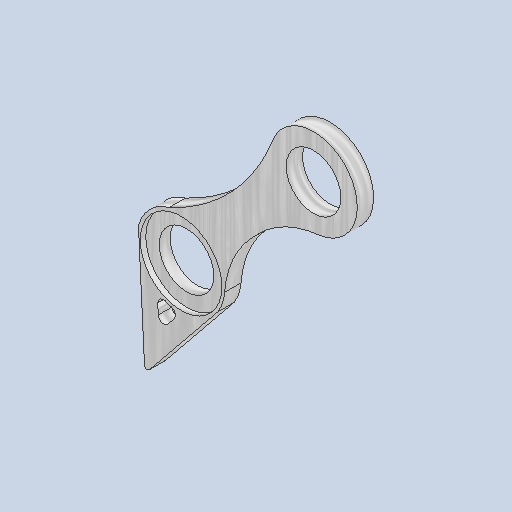
# Autodesk Inventor part: アーム 揺動節
Saved by Autodesk Inventor 2023 (Build 270158030, 158C)
## iProperties
Created: 2019-09-05
Part Number: アーム 揺動節
Material: アルミニウム 7075
Document SubType Name: Modeling
Designer: 雪村
Density: 2.81 g/cm^3
Appearance: サテン - ブラシ仕上げ 重厚
Mass: 3.77729 g
Surface Area: 16.4358 cm^2
Volume: 1.34423 cm^3
Description: アルミ2000 3t
Author: 雪村
Autodesk Inventor part; units mm, degrees
ref_plane "YZ Plane" through (0, 0, 0) normal (1, 0, 0) x (0, 1, 0)
ref_plane "XZ Plane" through (0, 0, 0) normal (0, 1, 0) x (-1, 0, 0)
ref_plane "XY Plane" through (0, 0, 0) normal (0, 0, 1) x (1, 0, 0)
sketch "スケッチ2" plane through (0, 0, 0) normal (0, 0, 1) x (1, 0, 0)
  circle A0 centre (-56.644, 91.4364) radius 8.025
  circle A1 centre (-56.644, 91.4364) radius 5.025
  arc A2 (-29.1424, 109.2011) -> (-49.1672, 88.5212) centre (-14.5297, 75.0161) ccw
  arc A3 (-59.7983, 98.8155) -> (-39.7735, 119.4954) centre (-74.411, 133.0005) ccw
  circle A4 centre (-32.2967, 116.5802) radius 8.025
  circle A5 centre (-32.2967, 116.5802) radius 5.025
  line L0 (-50.8789, 85.8539) -> (-64.3562, 71.9357)
  line L1 (-64.3562, 71.9357) -> (-64.668, 91.3073)
  line L2 (-56.644, 91.4364) -> (-32.2967, 116.5802) construction
  point P0 (0, 0)
  point P1 (0, 0)
  dimension "d5" = 45
  constraints: 6 centre point, 6 end point, 6 point on circle, 2 tangent, 1 parallel, 7 other
  measures "d5" angle of L0 L1
extrude "押し出し2" add sketch "スケッチ2" along normal blind 3
fillet "フィレット2" radius 0.5 1 edges at (-64.3562, 71.9357, 1.5)
sketch "スケッチ3" plane through (0, 0, 3) normal (0, 0, 1) x (1, 0, 0)
  line L0 (-63.5165, 72.8029) -> (-50.8789, 85.8539) projected
  arc A0 (-64.3756, 73.1427) -> (-63.5165, 72.8029) centre (-63.8757, 73.1507) ccw projected
  line L1 (-64.668, 91.3073) -> (-64.3756, 73.1427) projected
  arc A1 (-59.7983, 98.8155) -> (-64.668, 91.3073) centre (-56.644, 91.4364) ccw projected
  circle A2 centre (-56.644, 91.4364) radius 5.025 projected
  arc A3 (-50.8789, 85.8539) -> (-49.1672, 88.5212) centre (-56.644, 91.4364) ccw projected
  line L2 (-64.2129, 94.1033) -> (-63.8416, 71.0319)
  point P0 (0, 0)
  point P1 (-63.8676, 72.6508)
  dimension "d9" = 0.5
  constraints: 2 end point, 1 parallel, 1 point on circle
  measures "d9" distance between parallel lines of L1 L2
extrude "押し出し3" cut sketch "スケッチ3" against normal through all
fillet "フィレット3" radius 1 1 edges at (-63.8676, 72.6508, 1.5)
sketch "スケッチ4" plane through (0, 0, 3) normal (0, 0, 1) x (1, 0, 0)
  circle A0 centre (-56.644, 91.4364) radius 5.025 projected
  circle A1 centre (-32.2967, 116.5802) radius 5.025 projected
  arc A2 (-50.8789, 85.8539) -> (-49.1672, 88.5212) centre (-56.644, 91.4364) ccw projected
  line L0 (-50.8789, 85.8539) -> (-62.1849, 74.178) projected
  arc A3 (-63.9031, 74.8576) -> (-62.1849, 74.178) centre (-62.9033, 74.8737) ccw projected
  line L1 (-63.9031, 74.8576) -> (-64.2129, 94.1033) projected
  arc A4 (-59.7983, 98.8155) -> (-64.2129, 94.1033) centre (-56.644, 91.4364) ccw projected
  arc A5 (-59.7983, 98.8155) -> (-39.7735, 119.4954) centre (-74.411, 133.0005) ccw projected
  arc A6 (-29.1424, 109.2011) -> (-39.7735, 119.4954) centre (-32.2967, 116.5802) ccw projected
  arc A7 (-29.1424, 109.2011) -> (-49.1672, 88.5212) centre (-14.5297, 75.0161) ccw projected
  point P0 (0, 0)
sketch "スケッチ5" plane through (0, 0, 3) normal (0, 0, 1) x (1, 0, 0)
  circle A0 centre (-56.6451, 91.4352) radius 5.025
  circle A1 centre (-32.2979, 116.579) radius 5.025
  arc A2 (-50.2754, 86.5539) -> (-49.1683, 88.52) centre (-56.6451, 91.4352) ccw
  line L0 (-53.8399, 82.796) -> (-62.186, 74.1768)
  arc A3 (-63.9043, 74.8564) -> (-63.4923, 74.0635) centre (-62.9044, 74.8725) ccw
  line L1 (-63.9043, 74.8564) -> (-64.1215, 88.3503)
  arc A4 (-59.7994, 98.8143) -> (-64.4699, 93.2166) centre (-56.6451, 91.4352) ccw
  arc A5 (-59.7994, 98.8143) -> (-39.7746, 119.4942) centre (-74.4122, 132.9993) ccw
  arc A6 (-29.1436, 109.1999) -> (-39.7746, 119.4942) centre (-32.2979, 116.579) ccw
  arc A7 (-29.1436, 109.1999) -> (-49.1683, 88.52) centre (-14.5308, 75.0149) ccw
  line L2 (-83.3619, 46.2586) -> (-83.0117, 46.8656)
  arc A8 (-83.0117, 46.8656) -> (-84.2091, 48.3089) centre (-83.8778, 47.3654) ccw
  arc A9 (-84.8038, 48.1181) -> (-84.2091, 48.3089) centre (-88.0269, 59.1832) ccw
  arc A10 (-84.8038, 48.1181) -> (-85.306, 46.5345) centre (-84.5242, 47.158) ccw
  arc A11 (-85.0521, 46.1918) -> (-85.306, 46.5345) centre (-90.0169, 42.7785) ccw
  arc A12 (-85.0521, 46.1918) -> (-83.3619, 46.2586) centre (-84.2281, 46.7584) ccw
  arc A13 (-83.3002, 71.3425) -> (-83.1434, 69.6224) centre (-82.7197, 70.5282) ccw
  arc A14 (-76.5108, 59.6362) -> (-83.1434, 69.6224) centre (-88.0269, 59.1832) ccw
  arc A15 (-76.5108, 59.6362) -> (-74.7281, 59.0541) centre (-75.5116, 59.6755) ccw
  line L3 (-74.7281, 59.0541) -> (-66.7908, 69.0625)
  arc A16 (-66.7908, 69.0625) -> (-66.5756, 69.7348) centre (-67.5743, 69.6838) ccw
  line L4 (-66.5756, 69.7348) -> (-66.7153, 72.4721)
  arc A17 (-66.7153, 72.4721) -> (-67.8599, 73.4104) centre (-67.714, 72.4211) ccw
  arc A18 (-72.6132, 76.6262) -> (-67.8599, 73.4104) centre (-68.4798, 77.615) ccw
  arc A19 (-72.6132, 76.6262) -> (-73.9849, 77.3105) centre (-73.5858, 76.3936) ccw
  arc A20 (-73.9849, 77.3105) -> (-82.4826, 71.9828) centre (-60.5442, 46.4316) ccw
  arc A21 (-83.3002, 71.3425) -> (-82.4826, 71.9828) centre (-89.9903, 80.7269) ccw
  arc A22 (-110.8315, 31.539) -> (-109.4939, 30.5036) centre (-109.8361, 31.4432) ccw
  arc A23 (-101.7829, 26.9363) -> (-109.4939, 30.5036) centre (-107.4323, 24.8423) ccw
  arc A24 (-101.7829, 26.9363) -> (-100.1278, 26.5873) centre (-100.8452, 27.2839) ccw
  line L5 (-100.1278, 26.5873) -> (-91.546, 35.4257)
  arc A25 (-91.546, 35.4257) -> (-91.9436, 37.0698) centre (-92.2634, 36.1224) ccw
  arc A26 (-93.6931, 47.552) -> (-91.9436, 37.0698) centre (-90.0169, 42.7785) ccw
  arc A27 (-93.6931, 47.552) -> (-93.8022, 49.2096) centre (-94.3033, 48.3443) ccw
  arc A28 (-99.3351, 56.9581) -> (-93.8022, 49.2096) centre (-88.0269, 59.1832) ccw
  arc A29 (-99.3351, 56.9581) -> (-101.1863, 57.258) centre (-100.3162, 56.765) ccw
  line L6 (-101.1863, 57.258) -> (-106.2752, 48.2771)
  arc A30 (-106.2752, 48.2771) -> (-105.4755, 46.7866) centre (-105.4052, 47.7841) ccw
  arc A31 (-109.0024, 35.6122) -> (-105.4755, 46.7866) centre (-105.8991, 40.7765) ccw
  arc A32 (-109.0024, 35.6122) -> (-110.5128, 34.8508) centre (-109.5174, 34.755) ccw
  line L7 (-110.5128, 34.8508) -> (-110.8315, 31.539)
  circle A33 centre (-68.4798, 77.615) radius 1.25
  arc A34 (-64.1344, 80.7577) -> (-66.454, 82.6296) centre (-66.1318, 80.6557) ccw
  line L8 (-64.1344, 80.7577) -> (-63.5026, 68.3807)
  line L9 (-63.5026, 68.3807) -> (-76.8311, 51.5743)
  line L10 (-76.8311, 51.5743) -> (-83.9322, 39.2676)
  arc A35 (-84.9769, 37.8848) -> (-83.9322, 39.2676) centre (-90.0169, 42.7785) ccw
  line L11 (-84.9769, 37.8848) -> (-102.3922, 19.9486)
  arc A36 (-114.425, 25.5151) -> (-102.3922, 19.9486) centre (-107.4323, 24.8423) ccw
  line L12 (-114.425, 25.5151) -> (-112.8918, 41.4493)
  arc A37 (-112.0111, 44.2398) -> (-112.8918, 41.4493) centre (-105.8991, 40.7765) ccw
  line L13 (-112.0111, 44.2398) -> (-99.7723, 65.8386)
  arc A38 (-91.2432, 72.2945) -> (-99.7723, 65.8386) centre (-88.0269, 59.1832) ccw
  arc A39 (-91.2432, 72.2945) -> (-84.4369, 74.2589) centre (-89.9903, 80.7269) ccw
  arc A40 (-66.454, 82.6296) -> (-84.4369, 74.2589) centre (-60.5442, 46.4316) ccw
  circle A41 centre (-56.6793, 91.4683) radius 4
  circle A42 centre (-56.6793, 91.4683) radius 1.25
  circle A43 centre (-90.0169, 42.7785) radius 3.025
  circle A44 centre (-105.8991, 40.7765) radius 3.025
  circle A45 centre (-107.4323, 24.8423) radius 3.025
  circle A46 centre (-88.0269, 59.1832) radius 8.525
  circle A47 centre (-56.6793, 91.4683) radius 1.25
  line L14 (-32.2979, 116.579) -> (-56.6793, 91.4683)
  line L15 (-56.6793, 91.4683) -> (-88.0269, 59.1832)
  line L16 (-63.1972, 68.283) -> (-63.8347, 80.773)
  arc A48 (-63.8347, 80.773) -> (-66.5024, 82.9257) centre (-66.1318, 80.6557) ccw
  arc A49 (-66.5024, 82.9257) -> (-84.6323, 74.4865) centre (-60.5442, 46.4316) ccw
  arc A50 (-91.2565, 72.6) -> (-84.6323, 74.4865) centre (-89.9903, 80.7269) ccw
  arc A51 (-91.2565, 72.6) -> (-100.0334, 65.9865) centre (-88.0269, 59.1832) ccw
  line L17 (-100.0334, 65.9865) -> (-112.2721, 44.3877)
  arc A52 (-112.2721, 44.3877) -> (-113.1904, 41.4781) centre (-105.8991, 40.7765) ccw
  line L18 (-113.1904, 41.4781) -> (-114.7236, 25.5439)
  arc A53 (-114.7236, 25.5439) -> (-102.177, 19.7396) centre (-107.4323, 24.8423) ccw
  line L19 (-102.177, 19.7396) -> (-84.7616, 37.6758)
  arc A54 (-84.7616, 37.6758) -> (-83.6724, 39.1176) centre (-90.0169, 42.7785) ccw
  line L20 (-83.6724, 39.1176) -> (-76.5823, 51.4052)
  line L21 (-76.5823, 51.4052) -> (-63.1972, 68.283)
  arc A55 (-50.1385, 86.7434) -> (-64.1215, 88.3503) centre (-56.6793, 91.4683) ccw
  line L22 (-63.8347, 80.773) -> (-64.5039, 93.8831)
  line L23 (-76.8311, 51.5743) -> (-63.2204, 68.7366)
  circle A56 centre (-62.7886, 70.0857) radius 0.5
  line L24 (-62.3833, 69.7929) -> (-50.1385, 86.7434)
  line L25 (-63.5026, 68.3807) -> (-63.2204, 68.7366)
  line L26 (-62.3968, 69.775) -> (-61.9303, 70.3632)
  point P0 (0, 0)
  point P1 (0, 0)
  point P2 (0, 0)
  point P3 (-64.214, 94.1021)
  point P4 (-63.996, 83.9328)
  point P5 (-64.0495, 83.8777)
  point P6 (-64.2363, 88.6401)
  point P7 (-64.1215, 88.3503)
  point P8 (-50.2754, 86.5539)
  point P9 (-63.2879, 70.0602)
  point P10 (-64.0754, 85.487)
  point P11 (-58.8289, 99.2457)
  point P12 (-49.1573, 88.5483)
  point P13 (-64.012, 81.5482)
  point P14 (-64.485, 93.5124)
  dimension "d13" = 0.3
  dimension "d14" = 1
  constraints: 97 point on circle, 57 centre point, 54 end point, 6 point on line, 4 tangent, 1 coincident, 1 collinear, 16 other
  measures "d13" distance between parallel lines of L8 L16
  measures "d14" diameter of A56
extrude "押し出し4" cut sketch "スケッチ5" against normal blind 3 contours L22 A48 L1 L15 | L16 A3 L8 L1 A48 | L8 A3 L1
extrude "押し出し5" cut sketch "スケッチ5" against normal blind 3 contours A0 L15 A41 L14 | A0 L14 A55 L24 A56 L16 L22 L15 | L14 A41 L15 A0 | A0 L15 L22 L1 A55 A4 A5 L14 | L14 A42 L15 A41 | A41 L15 A42 L14 | L22 A48 L1 L15 | L15 L1 L22 | A2 L24 A55 | A5 A4 L22 A55 | L14 L15 A42 | A42 L15 L14 | L22 A55 L1 | L22 A55 | A56
extrude "押し出し6" add sketch "スケッチ5" against normal blind 3 contours A0 L14 A55 L24 A56 L16 L22 L15 | A0 L15 L22 L1 A55 A4 A5 L14 | A2 L24 A55 | A5 A4 L22 A55 | L22 A55 L1 | A56
sketch "スケッチ6" plane through (0, 0, 3) normal (0, 0, 1) x (1, 0, 0)
  arc A0 (-58.8326, 99.2446) -> (-39.7735, 119.4954) centre (-74.411, 133.0005) ccw projected
  arc A1 (-29.1424, 109.2011) -> (-39.7735, 119.4954) centre (-32.2967, 116.5802) ccw projected
  arc A2 (-29.1424, 109.2011) -> (-49.1672, 88.5212) centre (-14.5297, 75.0161) ccw projected
  circle A3 centre (-32.2967, 116.5802) radius 5.025 projected
  circle A4 centre (-56.6451, 91.4352) radius 5.025 projected
  arc A5 (-58.8326, 99.2446) -> (-64.485, 93.5124) centre (-56.6793, 91.4683) ccw projected
  arc A6 (-50.2787, 86.5493) -> (-49.1672, 88.5212) centre (-56.644, 91.4364) ccw projected
  line L0 (-50.2787, 86.5493) -> (-62.3833, 69.7929) projected
  arc A7 (-63.2879, 70.0602) -> (-62.3833, 69.7929) centre (-62.7886, 70.0857) ccw projected
  line L1 (-63.2879, 70.0602) -> (-64.485, 93.5124) projected
  point P0 (0, 0)
sketch "スケッチ7" plane through (0, 0, 3) normal (0, 0, 1) x (1, 0, 0)
  arc A0 (-58.8326, 99.2446) -> (-39.7735, 119.4954) centre (-74.411, 133.0005) ccw projected
  arc A1 (-29.1424, 109.2011) -> (-39.7735, 119.4954) centre (-32.2967, 116.5802) ccw projected
  arc A2 (-29.1424, 109.2011) -> (-49.1672, 88.5212) centre (-14.5297, 75.0161) ccw projected
  circle A3 centre (-32.2967, 116.5802) radius 5.025 projected
  circle A4 centre (-56.6451, 91.4352) radius 5.025 projected
  arc A5 (-58.8326, 99.2446) -> (-64.485, 93.5124) centre (-56.6793, 91.4683) ccw projected
  arc A6 (-50.2787, 86.5493) -> (-49.1672, 88.5212) centre (-56.644, 91.4364) ccw projected
  line L0 (-50.2787, 86.5493) -> (-62.3833, 69.7929) projected
  arc A7 (-63.2879, 70.0602) -> (-62.3833, 69.7929) centre (-62.7886, 70.0857) ccw projected
  line L1 (-63.2879, 70.0602) -> (-64.485, 93.5124) projected
  point P0 (0, 0)
sketch "スケッチ8" plane through (0, 0, 3) normal (0, 0, 1) x (1, 0, 0)
  circle A0 centre (-56.6451, 91.4352) radius 5.025 projected
  arc A1 (-58.8326, 99.2446) -> (-64.485, 93.5124) centre (-56.6793, 91.4683) ccw projected
  arc A2 (-58.8326, 99.2446) -> (-39.7735, 119.4954) centre (-74.411, 133.0005) ccw projected
  arc A3 (-29.1424, 109.2011) -> (-39.7735, 119.4954) centre (-32.2967, 116.5802) ccw projected
  arc A4 (-29.1424, 109.2011) -> (-49.1672, 88.5212) centre (-14.5297, 75.0161) ccw projected
  arc A5 (-50.2787, 86.5493) -> (-49.1672, 88.5212) centre (-56.644, 91.4364) ccw projected
  line L0 (-50.2787, 86.5493) -> (-62.3833, 69.7929) projected
  arc A6 (-63.2879, 70.0602) -> (-62.3833, 69.7929) centre (-62.7886, 70.0857) ccw projected
  line L1 (-63.2879, 70.0602) -> (-64.485, 93.5124) projected
  circle A7 centre (-32.2967, 116.5802) radius 5.025 projected
  line L2 (-56.644, 91.4364) -> (-32.2967, 116.5802)
  line L3 (-29.5619, 125.8734) -> (-71.0195, 83.0595)
  arc A8 (-58.8326, 99.2446) -> (-39.7735, 119.4954) centre (-74.411, 133.0005) ccw projected
  line L4 (-56.644, 91.4364) -> (-32.2967, 116.5802) construction
  line L5 (-55.2072, 90.0451) -> (-30.8599, 115.1889)
  line L6 (-33.7335, 117.9715) -> (-58.0808, 92.8277)
  arc A9 (-58.0808, 92.8277) -> (-55.2072, 90.0451) centre (-56.644, 91.4364) ccw
  arc A10 (-30.8599, 115.1889) -> (-33.7335, 117.9715) centre (-32.2967, 116.5802) ccw
  arc A11 (-29.1424, 109.2011) -> (-49.1672, 88.5212) centre (-14.5297, 75.0161) ccw projected
  circle A12 centre (-56.644, 91.4364) radius 8.025
  circle A13 centre (-32.2967, 116.5802) radius 8.025
  point P0 (0, 0)
  point P1 (-44.4704, 104.0083)
  point P2 (-36.2663, 109.6057)
  point P3 (-49.8009, 95.6283)
  dimension "d21" = 4.5
  dimension "d22" = 4
  constraints: 12 end point, 5 tangent, 4 point on circle, 2 centre point, 2 coincident, 2 parallel, 1 collinear, 1 midpoint, 6 other
  measures "d21" distance between parallel lines of L2 L3
  measures "d22" diameter of A10
extrude "押し出し7" cut sketch "スケッチ8" against normal blind 10 contours L5 A13 A4 A12
fillet "フィレット4" radius 18 2 edges at (-49.8009, 95.6283, 1.5) (-36.2663, 109.6057, 1.5)
sketch "スケッチ9" plane through (0, 0, 3) normal (0, 0, 1) x (1, 0, 0)
  circle A0 centre (-56.6451, 91.4352) radius 5.025 projected
  arc A1 (-58.8326, 99.2446) -> (-64.485, 93.5124) centre (-56.6793, 91.4683) ccw projected
  arc A2 (-58.8326, 99.2446) -> (-39.7735, 119.4954) centre (-74.411, 133.0005) ccw projected
  arc A3 (-31.4383, 108.6012) -> (-39.7735, 119.4954) centre (-32.2967, 116.5802) ccw projected
  arc A4 (-31.4383, 108.6012) -> (-42.4439, 103.226) centre (-29.5128, 90.7045) ccw projected
  line L0 (-42.4439, 103.226) -> (-43.6232, 102.0081) projected
  arc A5 (-43.6232, 102.0081) -> (-48.6415, 90.8352) centre (-30.6921, 89.4866) ccw projected
  arc A6 (-50.2787, 86.5493) -> (-48.6415, 90.8352) centre (-56.644, 91.4364) ccw projected
  line L1 (-50.2787, 86.5493) -> (-62.3833, 69.7929) projected
  arc A7 (-63.2879, 70.0602) -> (-62.3833, 69.7929) centre (-62.7886, 70.0857) ccw projected
  line L2 (-63.2879, 70.0602) -> (-64.485, 93.5124) projected
  circle A8 centre (-32.2967, 116.5802) radius 5.025 projected
  line L3 (-60.6541, 77.3098) -> (-52.682, 88.3456)
  arc A9 (-52.682, 88.3456) -> (-51.6331, 91.0599) centre (-56.644, 91.4364) ccw
  arc A10 (-45.7784, 104.095) -> (-51.6331, 91.0599) centre (-30.6921, 89.4866) ccw
  line L4 (-45.7784, 104.095) -> (-44.5991, 105.3129)
  arc A11 (-31.7592, 111.584) -> (-44.5991, 105.3129) centre (-29.5128, 90.7045) ccw
  arc A12 (-31.7592, 111.584) -> (-36.9785, 118.4056) centre (-32.2967, 116.5802) ccw
  arc A13 (-57.8274, 96.4055) -> (-36.9785, 118.4056) centre (-74.411, 133.0005) ccw
  arc A14 (-57.8274, 96.4055) -> (-61.4624, 93.1463) centre (-56.6793, 91.4683) ccw
  line L5 (-61.4624, 93.1463) -> (-60.6541, 77.3098)
  circle A15 centre (-56.644, 91.4364) radius 8.025
  point P0 (0, 0)
  point P1 (-56.239, 83.4216)
  point P2 (-61.0322, 84.7174)
  dimension "d26" = 3
  constraints: 12 point on circle, 6 centre point, 6 end point, 1 coincident, 11 other
  measures "d26" distance between parallel lines of L1 L3
extrude "押し出し8" cut sketch "スケッチ9" against normal blind 2.5 contours L3 L5 A15
fillet "フィレット5" radius 1 3 edges at (-61.0322, 84.7174, 1.75) (-56.239, 83.4216, 1.75) (-60.6541, 77.3098, 1.75)
sketch "スケッチ10" plane through (0, 0, 3) normal (0, 0, 1) x (1, 0, 0)
  line L0 (-60.799, 80.1484) -> (-60.9438, 82.9858) projected
  arc A0 (-59.5793, 83.9675) -> (-60.9438, 82.9858) centre (-59.9451, 83.0368) ccw projected
  arc A1 (-59.5793, 83.9675) -> (-57.9522, 83.5187) centre (-56.644, 91.4364) ccw projected
  arc A2 (-57.3045, 81.9465) -> (-57.9522, 83.5187) centre (-58.1152, 82.5321) ccw projected
  line L1 (-57.3045, 81.9465) -> (-58.9896, 79.6138) projected
  arc A3 (-60.799, 80.1484) -> (-58.9896, 79.6138) centre (-59.8003, 80.1994) ccw projected
  arc A4 (-31.4383, 108.6012) -> (-39.7735, 119.4954) centre (-32.2967, 116.5802) ccw projected
  arc A5 (-58.8326, 99.2446) -> (-39.7735, 119.4954) centre (-74.411, 133.0005) ccw projected
  arc A6 (-58.8326, 99.2446) -> (-64.485, 93.5124) centre (-56.6793, 91.4683) ccw projected
  line L2 (-64.485, 93.5124) -> (-63.2879, 70.0602) projected
  arc A7 (-63.2879, 70.0602) -> (-62.3833, 69.7929) centre (-62.7886, 70.0857) ccw projected
  line L3 (-62.3833, 69.7929) -> (-50.2787, 86.5493) projected
  arc A8 (-50.2787, 86.5493) -> (-48.6415, 90.8352) centre (-56.644, 91.4364) ccw projected
  arc A9 (-43.6232, 102.0081) -> (-48.6415, 90.8352) centre (-30.6921, 89.4866) ccw projected
  line L4 (-43.6232, 102.0081) -> (-42.4439, 103.226) projected
  arc A10 (-31.4383, 108.6012) -> (-42.4439, 103.226) centre (-29.5128, 90.7045) ccw projected
  circle A11 centre (-56.6451, 91.4352) radius 5.025 projected
  circle A12 centre (-32.2967, 116.5802) radius 5.025 projected
  circle A13 centre (-56.6451, 91.4352) radius 8.025
  point P0 (0, 0)
  dimension "d31" = 16.05
  constraints: 1 centre point, 1 coincident
  measures "d31" diameter of A13
sketch "スケッチ11" plane through (0, 0, 3) normal (0, 0, 1) x (1, 0, 0)
  line L0 (-61.9172, 97.5483) -> (-93.2211, 70.5805)
  arc A0 (-92.0093, 71.0583) -> (-93.2211, 70.5805) centre (-88.0269, 59.1832) ccw
  line L1 (-87.2798, 72.6443) -> (-92.0093, 71.0583)
  arc A1 (-87.2798, 72.6443) -> (-84.4369, 74.259) centre (-89.9903, 80.727) ccw
  arc A2 (-66.4541, 82.6296) -> (-84.4369, 74.259) centre (-60.5442, 46.4317) ccw
  arc A3 (-64.1344, 80.7577) -> (-66.4541, 82.6296) centre (-66.1318, 80.6558) ccw
  line L2 (-63.5959, 70.2078) -> (-64.1344, 80.7577)
  line L3 (-63.5959, 70.2078) -> (-50.4477, 86.412)
  arc A4 (-50.4477, 86.412) -> (-61.9172, 97.5483) centre (-56.6794, 91.4684) ccw
  circle A5 centre (-56.6794, 91.4684) radius 4
  line L4 (-60.799, 80.1484) -> (-60.9438, 82.9858) projected
  arc A6 (-59.5793, 83.9675) -> (-60.9438, 82.9858) centre (-59.9451, 83.0368) ccw projected
  arc A7 (-59.5793, 83.9675) -> (-57.9522, 83.5187) centre (-56.644, 91.4364) ccw projected
  arc A8 (-57.3045, 81.9465) -> (-57.9522, 83.5187) centre (-58.1152, 82.5321) ccw projected
  line L5 (-57.3045, 81.9465) -> (-58.9896, 79.6138) projected
  arc A9 (-60.799, 80.1484) -> (-58.9896, 79.6138) centre (-59.8003, 80.1994) ccw projected
  arc A10 (-31.4383, 108.6012) -> (-39.7735, 119.4954) centre (-32.2967, 116.5802) ccw projected
  arc A11 (-58.8326, 99.2446) -> (-39.7735, 119.4954) centre (-74.411, 133.0005) ccw projected
  arc A12 (-58.8326, 99.2446) -> (-64.485, 93.5124) centre (-56.6793, 91.4683) ccw projected
  line L6 (-64.485, 93.5124) -> (-63.2879, 70.0602) projected
  arc A13 (-63.2879, 70.0602) -> (-62.3833, 69.7929) centre (-62.7886, 70.0857) ccw projected
  line L7 (-62.3833, 69.7929) -> (-50.2787, 86.5493) projected
  arc A14 (-50.2787, 86.5493) -> (-48.6415, 90.8352) centre (-56.644, 91.4364) ccw projected
  arc A15 (-43.6232, 102.0081) -> (-48.6415, 90.8352) centre (-30.6921, 89.4866) ccw projected
  line L8 (-43.6232, 102.0081) -> (-42.4439, 103.226) projected
  arc A16 (-31.4383, 108.6012) -> (-42.4439, 103.226) centre (-29.5128, 90.7045) ccw projected
  circle A17 centre (-56.6451, 91.4352) radius 5.025 projected
  circle A18 centre (-32.2967, 116.5802) radius 5.025 projected
  line L9 (-50.4477, 86.412) -> (-49.8116, 87.196)
  line L10 (-62.3833, 69.7929) -> (-50.2787, 86.5493) projected
  point P0 (0, 0)
  point P1 (0, 0)
  point P2 (-49.8994, 87.0877)
  point P3 (-63.3132, 70.5562)
  constraints: 10 end point, 10 point on circle, 6 centre point, 1 collinear, 1 point on line, 63 other
extrude "押し出し9" cut sketch "スケッチ11" against normal blind 10 contours L9 A14 L7 A13 L6 L3
fillet "フィレット6" radius 0.5 1 edges at (-63.3132, 70.5562, 1.5)
sketch "スケッチ12" plane through (0, 0, 3) normal (0, 0, 1) x (1, 0, 0)
  line L0 (-60.799, 80.1484) -> (-60.9438, 82.9858) projected
  arc A0 (-59.5793, 83.9675) -> (-60.9438, 82.9858) centre (-59.9451, 83.0368) ccw projected
  arc A1 (-59.5793, 83.9675) -> (-57.9522, 83.5187) centre (-56.644, 91.4364) ccw projected
  arc A2 (-57.3045, 81.9465) -> (-57.9522, 83.5187) centre (-58.1152, 82.5321) ccw projected
  line L1 (-57.3045, 81.9465) -> (-58.9896, 79.6138) projected
  arc A3 (-60.799, 80.1484) -> (-58.9896, 79.6138) centre (-59.8003, 80.1994) ccw projected
  arc A4 (-63.3797, 71.8578) -> (-62.4921, 71.5682) centre (-62.8803, 71.8833) ccw projected
  line L2 (-62.4921, 71.5682) -> (-49.8994, 87.0877) projected
  arc A5 (-49.8994, 87.0877) -> (-48.6415, 90.8352) centre (-56.644, 91.4364) ccw projected
  arc A6 (-43.6232, 102.0081) -> (-48.6415, 90.8352) centre (-30.6921, 89.4866) ccw projected
  line L3 (-43.6232, 102.0081) -> (-42.4439, 103.226) projected
  arc A7 (-31.4383, 108.6012) -> (-42.4439, 103.226) centre (-29.5128, 90.7045) ccw projected
  arc A8 (-31.4383, 108.6012) -> (-39.7735, 119.4954) centre (-32.2967, 116.5802) ccw projected
  arc A9 (-58.8326, 99.2446) -> (-39.7735, 119.4954) centre (-74.411, 133.0005) ccw projected
  arc A10 (-58.8326, 99.2446) -> (-64.485, 93.5124) centre (-56.6793, 91.4683) ccw projected
  line L4 (-64.485, 93.5124) -> (-63.3797, 71.8578) projected
  circle A11 centre (-56.6451, 91.4352) radius 5.025 projected
  circle A12 centre (-32.2967, 116.5802) radius 5.025 projected
  line L5 (-52.3441, 88.8361) -> (-60.7158, 78.5186)
  line L6 (-60.7158, 78.5186) -> (-61.4624, 93.1463)
  arc A13 (-57.8274, 96.4055) -> (-61.4624, 93.1463) centre (-56.6793, 91.4683) ccw
  arc A14 (-57.8274, 96.4055) -> (-36.9785, 118.4056) centre (-74.411, 133.0005) ccw
  arc A15 (-31.7592, 111.584) -> (-36.9785, 118.4056) centre (-32.2967, 116.5802) ccw
  arc A16 (-31.7592, 111.584) -> (-44.5991, 105.3129) centre (-29.5128, 90.7045) ccw
  line L7 (-44.5991, 105.3129) -> (-45.7784, 104.095)
  arc A17 (-45.7784, 104.095) -> (-51.6331, 91.0599) centre (-30.6921, 89.4866) ccw
  arc A18 (-52.3441, 88.8361) -> (-51.6331, 91.0599) centre (-56.644, 91.4364) ccw
  point P0 (0, 0)
  point P1 (-57.1774, 82.8794)
  point P2 (-60.1206, 79.2521)
  dimension "d35" = 3
  constraints: 12 point on circle, 6 centre point, 6 end point, 8 other
  measures "d35" distance between parallel lines of L2 L5
extrude "押し出し10" add sketch "スケッチ12" against normal blind 3 contours L5 A2 L1 A3
fillet "フィレット7" radius 1 2 edges at (-60.1206, 79.2521, 1.75) (-57.1774, 82.8794, 1.75)
sketch "スケッチ13" plane through (0, 0, 3) normal (0, 0, 1) x (1, 0, 0)
  arc A0 (-57.8834, 82.0093) -> (-58.4365, 83.6142) centre (-58.6599, 82.6394) ccw projected
  line L0 (-57.8834, 82.0093) -> (-59.0734, 80.5427) projected
  arc A1 (-60.8486, 81.1218) -> (-59.0734, 80.5427) centre (-59.8499, 81.1728) ccw projected
  line L1 (-60.8486, 81.1218) -> (-60.9438, 82.9858) projected
  arc A2 (-59.5793, 83.9675) -> (-60.9438, 82.9858) centre (-59.9451, 83.0368) ccw projected
  arc A3 (-59.5793, 83.9675) -> (-58.4365, 83.6142) centre (-56.644, 91.4364) ccw projected
  arc A4 (-63.3797, 71.8578) -> (-62.4921, 71.5682) centre (-62.8803, 71.8833) ccw projected
  line L2 (-62.4921, 71.5682) -> (-49.8994, 87.0877) projected
  arc A5 (-49.8994, 87.0877) -> (-48.6415, 90.8352) centre (-56.644, 91.4364) ccw projected
  arc A6 (-43.6232, 102.0081) -> (-48.6415, 90.8352) centre (-30.6921, 89.4866) ccw projected
  line L3 (-43.6232, 102.0081) -> (-42.4439, 103.226) projected
  arc A7 (-31.4383, 108.6012) -> (-42.4439, 103.226) centre (-29.5128, 90.7045) ccw projected
  arc A8 (-31.4383, 108.6012) -> (-39.7735, 119.4954) centre (-32.2967, 116.5802) ccw projected
  arc A9 (-58.8326, 99.2446) -> (-39.7735, 119.4954) centre (-74.411, 133.0005) ccw projected
  arc A10 (-58.8326, 99.2446) -> (-64.485, 93.5124) centre (-56.6793, 91.4683) ccw projected
  line L4 (-64.485, 93.5124) -> (-63.3797, 71.8578) projected
  circle A11 centre (-56.6451, 91.4352) radius 5.025 projected
  circle A12 centre (-32.2967, 116.5802) radius 5.025 projected
  circle A13 centre (-56.6451, 91.4352) radius 7.5
  point P0 (0, 0)
  dimension "d39" = 15
  constraints: 1 centre point, 1 coincident
  measures "d39" diameter of A13
extrude "押し出し11" cut sketch "スケッチ13" against normal blind 1 contours A13
